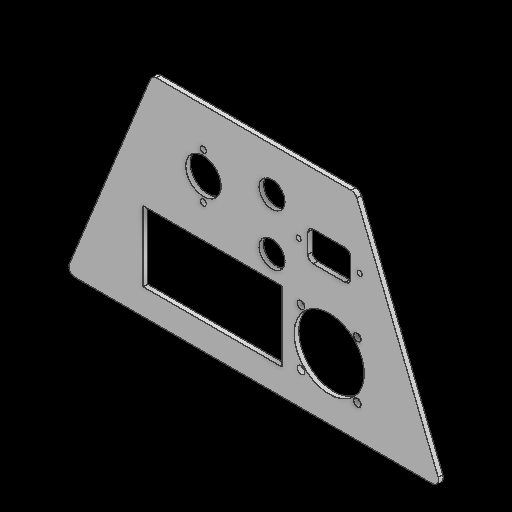
# Autodesk Inventor part: BreakerMount
Saved by Autodesk Inventor 2025.2 (Build 292293000, 293)
## iProperties
Created: 2025-11-18
Part Number: BreakerMount
Material: Generic
Document SubType Name: Sheet Metal
Designer: valer
Density: 1 g/cm^3
Sheet Metal Rule: Default
Appearance: Default
Author: valer
Autodesk Inventor part; units mm, degrees
ref_plane "YZ Plane" through (0, 0, 0) normal (1, 0, 0) x (0, 1, 0)
ref_plane "XZ Plane" through (0, 0, 0) normal (0, 1, 0) x (-1, 0, 0)
ref_plane "XY Plane" through (0, 0, 0) normal (0, 0, 1) x (1, 0, 0)
sketch "Base" plane through (0, 0, 0) normal (0, 0, 1) x (1, 0, 0)
  line L0 (0, 0) -> (70.3402, 0)
  line L1 (70.3402, 0) -> (142.1613, -140)
  line L2 (142.1613, -140) -> (0, -140)
  line L3 (0, -140) -> (0, 0) construction
  line L4 (0, 0) -> (-70.3402, 0)
  line L5 (-70.3402, 0) -> (-142.1613, -140)
  line L6 (-142.1613, -140) -> (0, -140)
  line L7 (-63.3831, 22.3248) -> (-182.4251, -209.7225) construction
  dimension "d1" = 140
  dimension "d3" = 4
  measures "d1" distance between parallel lines of L6 L4
  measures "d3" distance between parallel lines of L7 L5
extrude "Plate1" add sketch "Base" along normal blind 3
fillet "FilletsFeature" radius 6 4 edges at (-70.3402, 0, 1.5) (70.3402, 0, 1.5) (142.1613, -140, 1.5) (-142.1613, -140, 1.5)
sketch "MatchProduction" plane through (0, 0, 3) normal (0, 0, 1) x (1, 0, 0)
  line L0 (0, -168.1502) -> (0, 28.901) construction
  line L1 (-66.6748, 0) -> (66.6748, 0) projected
  line L2 (66.6748, 0) -> (123.2385, -140)
  line L3 (132.3398, -140) -> (-132.3398, -140) projected
  arc A0 (72.0133, -3.2613) -> (66.6748, 0) centre (66.6748, -6) ccw projected
  line L4 (72.0133, -3.2613) -> (137.6783, -131.2613) projected
  arc A1 (132.3398, -140) -> (137.6783, -131.2613) centre (132.3398, -134) ccw projected
  arc A2 (-137.6783, -131.2613) -> (-132.3398, -140) centre (-132.3398, -134) ccw projected
  line L5 (-137.6783, -131.2613) -> (-72.0133, -3.2613) projected
  arc A3 (-66.6748, 0) -> (-72.0133, -3.2613) centre (-66.6748, -6) ccw projected
  line L6 (-66.6748, 0) -> (-123.2385, -140)
  point P0 (0, 0)
  point P1 (-123.2385, -140)
  dimension "d13" = 68
  constraints: 4 end point, 1 point on line, 1 symmetric about line
  measures "d13" angle of L3 L2
extrude "MatchProductionFeature" cut sketch "MatchProduction" against normal blind 3 contours L6 L3 A2 L5 A3 | A0 L4 A1 L3 L2
fillet "OutsideFilletsFeature" radius 4 4 edges at (-123.2385, -140, 1.5) (123.2385, -140, 1.5) (66.6748, 0, 1.5) (-66.6748, 0, 1.5)
sketch "PanelControls" plane through (0, 0, 0) normal (0, 0, -1) x (-1, 0, 0)
  circle A0 centre (33, -55.3581) radius 2 projected
  circle A1 centre (33, -25.3581) radius 2 projected
  circle A2 centre (-12, -62.1443) radius 8 projected
  circle A3 centre (-12, -28.2391) radius 8 projected
  line L0 (72, -122.5) -> (72, -77.5) construction
  line L1 (18, -122.5) -> (72, -122.5) construction
  line L2 (72, -77.5) -> (18, -77.5) construction
  line L3 (18, -77.5) -> (18, -122.5) construction
  line L4 (18, -77.5) -> (0.05, -77.5) construction
  line L5 (0.05, -122.5) -> (18, -122.5) construction
  circle A4 centre (-31, -81.5) radius 2.5 projected
  circle A5 centre (-31, -118.5) radius 2.5 projected
  circle A6 centre (-68, -118.5) radius 2.5 projected
  circle A7 centre (-68, -81.5) radius 2.5 projected
  circle A8 centre (-29.5, -44.3793) radius 1.65 projected
  circle A9 centre (-69.5, -44.3793) radius 1.65 projected
  circle A10 centre (-49.5, -100) radius 22.5 projected
  arc A11 (33, -51.4831) -> (33, -29.2331) centre (33, -40.3581) ccw projected
  line L6 (-38.95, -53.7293) -> (-60.05, -53.7293) projected
  arc A12 (-38.95, -53.7293) -> (-35.95, -50.7293) centre (-38.95, -50.7293) ccw projected
  line L7 (-35.95, -38.0293) -> (-35.95, -50.7293) projected
  arc A13 (-35.95, -38.0293) -> (-38.95, -35.0293) centre (-38.95, -38.0293) ccw projected
  line L8 (-60.05, -35.0293) -> (-38.95, -35.0293) projected
  arc A14 (-60.05, -35.0293) -> (-63.05, -38.0293) centre (-60.05, -38.0293) ccw projected
  line L9 (-63.05, -50.7293) -> (-63.05, -38.0293) projected
  arc A15 (-63.05, -50.7293) -> (-60.05, -53.7293) centre (-60.05, -50.7293) ccw projected
  arc A16 (33, -51.4831) -> (33, -29.2331) centre (33, -40.3581) ccw projected
  circle A17 centre (33, -40.3581) radius 11.125 projected
  line L10 (-0.05, -77.5) -> (-18, -77.5) construction
  line L11 (-18, -78.5) -> (-18, -121.5) construction
  line L12 (-18, -122.5) -> (-0.05, -122.5) construction
  line L13 (0.05, -122.5) -> (18, -122.5) construction
  line L14 (-18, -122.5) -> (-18, -121.5) construction
  line L15 (-18, -78.5) -> (-18, -77.5) construction
  line L16 (-18, -77.5) -> (72, -77.5)
  line L17 (72, -77.5) -> (72, -122.5)
  line L18 (72, -122.5) -> (-18, -122.5)
  line L19 (-18, -122.5) -> (-18, -77.5)
  point P0 (0, 0)
  constraints: 12 end point, 2 parallel, 2 vertical, 1 horizontal, 1 perpendicular
extrude "PanelControlsFeature" cut sketch "PanelControls" against normal blind 3
sketch "PanelControlsExpand" plane through (0, 0, 0) normal (0, 0, -1) x (-1, 0, 0)
  line L0 (-60.05, -35.0293) -> (-38.95, -35.0293) projected
  arc A0 (-60.05, -35.0293) -> (-63.05, -38.0293) centre (-60.05, -38.0293) ccw projected
  line L1 (-63.05, -50.7293) -> (-63.05, -38.0293) projected
  line L2 (-35.95, -38.0293) -> (-35.95, -50.7293) projected
  arc A1 (-35.95, -38.0293) -> (-38.95, -35.0293) centre (-38.95, -38.0293) ccw projected
  arc A2 (-38.95, -53.7293) -> (-35.95, -50.7293) centre (-38.95, -50.7293) ccw projected
  line L3 (-38.95, -53.7293) -> (-60.05, -53.7293) projected
  arc A3 (-63.05, -50.7293) -> (-60.05, -53.7293) centre (-60.05, -50.7293) ccw projected
  circle A4 centre (-12, -28.2391) radius 8 projected
  circle A5 centre (-12, -62.1443) radius 8 projected
  circle A6 centre (33, -40.3581) radius 11.125 projected
  circle A7 centre (-49.5, -100) radius 22.5 projected
  line L4 (-18, -77.5) -> (72, -77.5) projected
  line L5 (-18, -122.5) -> (-18, -77.5) projected
  line L6 (72, -122.5) -> (-18, -122.5) projected
  line L7 (72, -77.5) -> (72, -122.5) projected
  line L8 (-38.95, -34.5293) -> (-60.05, -34.5293)
  arc A8 (-60.05, -34.5293) -> (-63.55, -38.0293) centre (-60.05, -38.0293) ccw
  line L9 (-63.55, -38.0293) -> (-63.55, -50.7293)
  arc A9 (-63.55, -50.7293) -> (-60.05, -54.2293) centre (-60.05, -50.7293) ccw
  line L10 (-60.05, -54.2293) -> (-38.95, -54.2293)
  arc A10 (-38.95, -54.2293) -> (-35.45, -50.7293) centre (-38.95, -50.7293) ccw
  line L11 (-35.45, -50.7293) -> (-35.45, -38.0293)
  arc A11 (-35.45, -38.0293) -> (-38.95, -34.5293) centre (-38.95, -38.0293) ccw
  circle A12 centre (-12, -28.2391) radius 8.5
  circle A13 centre (33, -40.3581) radius 11.625
  circle A14 centre (-12, -62.1443) radius 8.5
  circle A15 centre (-49.5, -100) radius 23
  line L12 (72.5, -77) -> (-18.5, -77)
  line L13 (-18.5, -77) -> (-18.5, -123)
  line L14 (-18.5, -123) -> (72.5, -123)
  line L15 (72.5, -123) -> (72.5, -77)
  point P0 (0, 0)
  dimension "d19" = 0.5
  dimension "d20" = 0.5
  dimension "d21" = 0.5
  dimension "d22" = 0.5
  dimension "d23" = 0.5
  dimension "d24" = 0.5
  constraints: 16 end point, 8 centre point, 8 point on circle, 10 other
  measures "d19" distance between parallel lines of L0 L8
  measures "d20" radial gap between concentric circles of A4 A12
  measures "d21" radial gap between concentric circles of A6 A13
  measures "d22" radial gap between concentric circles of A5 A14
  measures "d23" radial gap between concentric circles of A7 A15
  measures "d24" distance between parallel lines of L4 L12
extrude "PanelControlsExpandFeature" cut sketch "PanelControlsExpand" against normal blind 3 contours L0 A1 L2 A2 L3 A3 L1 A0 | A4 | A5 | A6 | A7 | L4 L7 L6 L5 | A11 L11 A10 L10 A9 L9 A8 L8 | A12 | A13 | A14 | A15 | L15 L14 L13 L12
equation "\"d14\" = Thickness"
equation "\"d17\" = Thickness"
equation "\"d25\" = Thickness"
equation "\"d0\" = Thickness"
equation "\"BendRadius\" = Thickness"
equation "\"BendReliefWidth\" = Thickness"
equation "\"BendReliefDepth\" = 0.5 * Thickness"
equation "\"CornerReliefSize\" = 4 * Thickness"
equation "\"MinimumRemnant\" = 2 * Thickness"
equation "\"TransitionRadius\" = BendRadius"
equation "\"JacobiRadiusSize\" = BendRadius"
equation "\"GapSize\" = Thickness"
equation "\"Thickness\" = 3"
body "Solid1"
